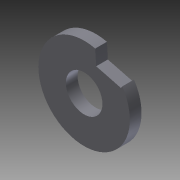
# Autodesk Inventor part: Gear Washer Spacer 3
Saved by Autodesk Inventor 2014 SP1 (Build 180222100, 222)
## iProperties
Created: 2012-03-30
Part Number: Gear Washer Spacer 3
Material: Steel
Document SubType Name: Modeling
Designer: Moses
Mass: 2.51195 g
Surface Area: 4.60053 cm^2
Volume: 0.319994 cm^3
Density: 7.85 g/cm^3
Appearance: Steel
Author: Moses
Autodesk Inventor part; units mm, degrees
ref_plane "YZ Plane" through (0, 0, 0) normal (1, 0, 0) x (0, 1, 0)
ref_plane "XZ Plane" through (0, 0, 0) normal (0, 1, 0) x (-1, 0, 0)
ref_plane "XY Plane" through (0, 0, 0) normal (0, 0, 1) x (1, 0, 0)
sketch "Sketch1" plane through (0, 0, 0) normal (0, 0, 1) x (1, 0, 0)
  circle A0 centre (0, 0) radius 7.9375
  circle A1 centre (0, 0) radius 3.175
  dimension "d0" = 15.875
  dimension "d1" = 6.35
  constraints: 2 centre point, 2 coincident
  measures "d0" diameter of A0
  measures "d1" diameter of A1
extrude "Extrusion1" add sketch "Sketch1" along normal blind 2.032
sketch "Sketch2" plane through (0, 0, 2.032) normal (0, 0, 1) x (1, 0, 0)
  circle A0 centre (0, 0) radius 7.9375 construction
  arc A1 (2.0793, 5.1162) -> (0.2784, 17.7544) centre (-62.2212, 2.4011) ccw projected
  arc A2 (14.1052, 14.1744) -> (6.3972, 3.9982) centre (61.3005, -29.5808) ccw projected
  arc A3 (6.3972, 3.9982) -> (2.0793, 5.1162) centre (-39.8868, -165.864) ccw projected
  arc A4 (6.6263, 4.3699) -> (1.9179, 7.7023) centre (0, 0) ccw
  constraints: 4 point on circle, 1 centre point, 1 coincident, 1 concentric
extrude "Extrusion2" cut sketch "Sketch2" against normal blind 25.4
body "Solid1"
